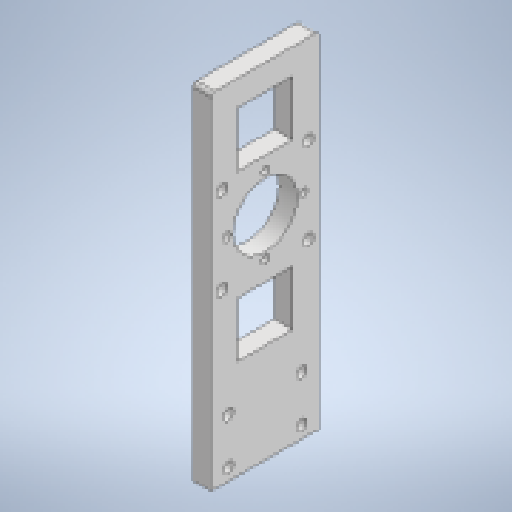
# Autodesk Inventor part: Y_Gantry_Connector
Saved by Autodesk Inventor 2023 (Build 270158000, 158)
## iProperties
Created: 2022-04-30
Part Number: Y_Gantry_Connector
Material: Generic
Document SubType Name: Modeling
Designer: plebbb
Density: 1 g/cm^3
Appearance: Default
Author: plebbb
Autodesk Inventor part; units mm, degrees
ref_plane "YZ Plane" through (0, 0, 0) normal (1, 0, 0) x (0, 1, 0)
ref_plane "XZ Plane" through (0, 0, 0) normal (0, 1, 0) x (-1, 0, 0)
ref_plane "XY Plane" through (0, 0, 0) normal (0, 0, 1) x (1, 0, 0)
sketch "Sketch1" plane through (0, 0, 0) normal (1, 0, 0) x (0, 1, 0)
  circle A0 centre (31.6, -9.4) radius 3
  circle A1 centre (31.6, -49.4) radius 3
  circle A2 centre (6.6, -9.4) radius 3
  circle A3 centre (6.6, -49.4) radius 3
  line L0 (31.6, -9.4) -> (6.6, -9.4) construction
  line L1 (6.6, -9.4) -> (6.6, -49.4) construction
  line L2 (6.6, -49.4) -> (31.6, -49.4) construction
  line L3 (31.6, -49.4) -> (31.6, -9.4) construction
  line L4 (0, 0) -> (38.2, 0)
  line L5 (38.2, 0) -> (38.2, -58.8)
  line L6 (38.2, -58.8) -> (0, -58.8)
  line L7 (0, -58.8) -> (0, 0)
  point P0 (31.6, -29.4)
  point P1 (38.2, -29.4)
  point P2 (19.1, -49.4)
  point P3 (19.1, -58.8)
  dimension "d0" = 6
  dimension "d1" = 25
  dimension "d2" = 40
  dimension "d3" = 58.8
  dimension "d4" = 38.2
  constraints: 16 end point, 5 coincident, 4 centre point, 4 midpoint, 4 parallel, 3 equal radius, 2 horizontal, 2 perpendicular, 1 horizontal alignment, 1 vertical alignment
  measures "d0" diameter of A0
  measures "d1" distance of L1.end L2.end
  measures "d2" distance of L2.end L0.start
  measures "d3" distance of L4.end L5.end
  measures "d4" distance of L5.end L6.end
extrude "Extrusion1" add sketch "Sketch1" along normal blind 10
sketch "Sketch3" plane through (10, 0, 0) normal (1, 0, 0) x (0, 0, -1)
  line L0 (58.8, 38.2) -> (0, 38.2) projected
  line L1 (0, 38.2) -> (0, 186.2)
  line L2 (2, 188.2) -> (56.8, 188.2)
  line L3 (58.8, 186.2) -> (58.8, 38.2)
  arc A0 (2, 188.2) -> (0, 186.2) centre (2, 186.2) ccw
  arc A1 (58.8, 186.2) -> (56.8, 188.2) centre (56.8, 186.2) ccw
  line L4 (14.4, 174.2) -> (44.4, 174.2)
  line L5 (44.4, 174.2) -> (44.4, 144.2)
  line L6 (44.4, 144.2) -> (14.4, 144.2)
  line L7 (14.4, 144.2) -> (14.4, 174.2)
  line L8 (14.4, 84.2) -> (44.4, 84.2)
  line L9 (44.4, 84.2) -> (44.4, 54.2)
  line L10 (44.4, 54.2) -> (14.4, 54.2)
  line L11 (14.4, 54.2) -> (14.4, 84.2)
  point P0 (0, 0)
  point P1 (29.4, 38.2)
  point P2 (29.4, 174.2)
  point P3 (29.4, 84.2)
  point P4 (29.4, 188.2)
  point P5 (29.4, 38.2)
  point P6 (29.4, 54.2)
  point P7 (29.4, 38.2)
  dimension "d7" = 150
  dimension "d8" = 2
  dimension "d9" = 30
  dimension "d12" = 60
  dimension "d13" = 16
  constraints: 22 end point, 7 midpoint, 6 perpendicular, 4 parallel, 4 point on circle, 4 tangent, 2 centre point, 2 horizontal, 2 vertical, 2 vertical alignment, 1 equal radius, 1 point on line
  measures "d7" distance from line of point (29.4, 38.2) L2
  measures "d8" radius of A0
  measures "d9" distance of L4.start L4.end
  measures "d12" distance from line of point (29.4, 84.2) L6
  measures "d13" distance of point (29.4, 54.2) point (29.4, 38.2)
extrude "Extrusion2" add sketch "Sketch3" against normal blind 10
sketch "Sketch4" plane through (0, 0, 0) normal (-1, 0, 0) x (0, 0, 1)
  circle A0 centre (-52.97, 139.57) radius 3
  circle A1 centre (-5.83, 139.57) radius 3
  circle A2 centre (-52.97, 92.43) radius 3
  circle A3 centre (-5.83, 92.43) radius 3
  line L0 (-52.97, 92.43) -> (-5.83, 92.43) construction
  line L1 (-5.83, 92.43) -> (-5.83, 139.57) construction
  line L2 (-5.83, 139.57) -> (-52.97, 139.57) construction
  line L3 (-52.97, 139.57) -> (-52.97, 92.43) construction
  line L4 (-57.6, 87.8) -> (-1.2, 87.8) construction
  line L5 (-1.2, 87.8) -> (-1.2, 144.2) construction
  line L6 (-1.2, 144.2) -> (-57.6, 144.2) construction
  line L7 (-57.6, 144.2) -> (-57.6, 87.8) construction
  line L8 (-14.4, 144.2) -> (-44.4, 144.2) construction
  circle A4 centre (-29.4, 116) radius 17.5
  line L9 (-8.4, 116) -> (-29.4, 137) construction
  line L10 (-29.4, 137) -> (-50.4, 116) construction
  line L11 (-50.4, 116) -> (-29.4, 95) construction
  line L12 (-29.4, 95) -> (-8.4, 116) construction
  circle A5 centre (-29.4, 137) radius 2.25
  circle A6 centre (-50.4, 116) radius 2.25
  circle A7 centre (-8.4, 116) radius 2.25
  circle A8 centre (-29.4, 95) radius 2.25
  point P0 (0, 0)
  point P1 (-1.2, 116)
  point P2 (-5.83, 116)
  point P3 (-29.4, 139.57)
  point P4 (-29.4, 144.2)
  point P5 (-29.4, 144.2)
  dimension "d16" = 47.14
  dimension "d17" = 6
  dimension "d18" = 56.4
  dimension "d19" = 35
  dimension "d22" = 42
  dimension "d23" = 4.5
  constraints: 24 end point, 9 centre point, 9 coincident, 8 perpendicular, 6 equal radius, 6 midpoint, 4 parallel, 4 vertical alignment, 3 horizontal alignment, 2 horizontal
  measures "d16" distance of L1.end L2.end
  measures "d17" diameter of A1
  measures "d18" distance of L5.end L6.end
  measures "d19" diameter of A4
  measures "d22" distance of L11.end L9.end
  measures "d23" diameter of A5
extrude "Extrusion3" cut sketch "Sketch4" against normal up to surface (10 mm away)
body "Solid1"
